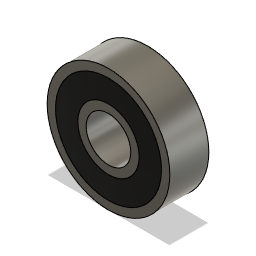
608 Bearings v1 (Autodesk Fusion 360 design; units mm, degrees)
Autodesk Fusion 360 part; units mm, degrees
sketch "Sketch1" plane through (0, 0, 0) normal (0, 0, 1) x (1, 0, 0)
  circle A0 centre (0, 0) radius 11
  circle A1 centre (0, 0) radius 9.5
  circle A2 centre (0, 0) radius 4
  circle A3 centre (0, 0) radius 5.5
  dimension "d1" = 22
  dimension "d2" = -1.5
  dimension "d3" = 8
  dimension "d4" = 1.5
  constraint coincident A0.centre A1.centre
  measures "d1" diameter of A0
  measures "d3" diameter of A2
extrude "Extrude1" add sketch "Sketch1" along normal blind 7 makes body 1 at (5.4727, -0.5476, 4.6667) makes body 2 at (10.9453, -1.0952, 4.6667)
extrude "Extrude2" add sketch "Sketch1" along normal blind 7 separate body contours A1 makes body 3
